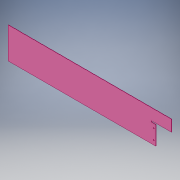
# Autodesk Inventor part: X-Axis Panel Left
Saved by Autodesk Inventor 2018 (Build 220112000, 112)
## iProperties
Created: 2018-10-23
Part Number: X-Axis Panel Left
Material: Steel
Document SubType Name: Modeling
Designer: P301319
Density: 7.85 g/cm^3
Appearance: Pink
Author: P301319
Autodesk Inventor part; units mm, degrees
ref_plane "YZ Plane" through (0, 0, 0) normal (1, 0, 0) x (0, 1, 0)
ref_plane "XZ Plane" through (0, 0, 0) normal (0, 1, 0) x (-1, 0, 0)
ref_plane "XY Plane" through (0, 0, 0) normal (0, 0, 1) x (1, 0, 0)
sketch "Sketch1" plane through (0, 0, 0) normal (0, 1, 0) x (-1, 0, 0)
  line L0 (0, 0) -> (-710, 0)
  line L1 (-710, 0) -> (-710, -150)
  line L2 (-710, -150) -> (0, -150)
  line L3 (0, -150) -> (0, 0)
  dimension "d0" = 710
  dimension "d1" = 150
  constraints: 8 end point, 2 parallel, 1 horizontal, 1 perpendicular
  measures "d0" distance of L2.end L1.end
  measures "d1" distance of L1.end L0.end
extrude "Extrusion1" add sketch "Sketch1" along normal blind 1.6
sketch "Sketch2" plane through (0, 1.6, 0) normal (0, 1, 0) x (1, 0, 0)
  line L0 (710, 0) -> (690, 0)
  line L1 (690, 0) -> (690, 60)
  line L2 (690, 60) -> (710, 60)
  line L3 (710, 60) -> (710, 0)
  circle A0 centre (700, 80) radius 2.5
  circle A1 centre (700, 130) radius 2.5
  line L4 (710, 150) -> (0, 150) projected
  point P0 (0, 0)
  point P1 (700, 60)
  dimension "d6" = 20
  dimension "d7" = 60
  dimension "d10" = 5
  dimension "d11" = 5
  dimension "d12" = 50
  dimension "d13" = 20
  constraints: 8 end point, 2 centre point, 2 parallel, 2 vertical alignment, 1 horizontal, 1 midpoint, 1 perpendicular
  measures "d6" distance of L1.end L2.end
  measures "d7" distance of L0.end L1.end
  measures "d10" diameter of A0
  measures "d11" diameter of A1
  measures "d12" distance of A0.centre A1.centre
  measures "d13" distance from line of L4 A1.centre
extrude "Extrusion3" cut sketch "Sketch2" against normal blind 1.6
sketch "Sketch3" plane through (690, 1.6, 0) normal (1, 0, 0) x (0, 0, -1)
  line L0 (0, -1.6) -> (54, -1.6)
  line L1 (54, -1.6) -> (54, 0)
  line L2 (54, 0) -> (0, 0)
  line L3 (0, 0) -> (0, -1.6)
  dimension "d16" = 54
  dimension "d17" = 1.6
  constraints: 8 end point, 2 parallel, 1 horizontal, 1 perpendicular
  measures "d16" distance of L2.end L1.end
  measures "d17" distance of L1.end L0.end
extrude "Extrusion4" add sketch "Sketch3" along normal blind 95
body "Solid1"
